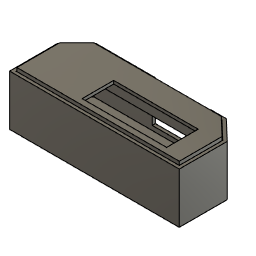
humid_atmega328p v1 (Autodesk Fusion 360 design; units mm, degrees)
Autodesk Fusion 360 part; units mm, degrees
sketch "base" plane through (0, 0, 0) normal (0, 1, 0) x (1, 0, 0)
  line L0 (-25.5013, -7.5251) -> (-25.5013, -7.5251)
  line L1 (26.2751, 6.2603) -> (26.2751, -7.5251)
  line L2 (26.2751, -7.5251) -> (-25.5249, -7.5251)
  line L3 (-25.5249, -7.5251) -> (-25.5249, 6.2605)
  line L4 (-25.5249, 6.2605) -> (-20.01, 11.7751)
  line L5 (-20.01, 11.7751) -> (20.5096, 11.7751)
  line L6 (20.5096, 11.7751) -> (20.5136, 11.771)
  line L7 (20.5136, 11.771) -> (20.5142, 11.771)
  line L8 (20.5142, 11.771) -> (26.2751, 6.2603)
  line L9 (27.2751, 6.6876) -> (27.2751, -8.5251)
  line L10 (27.2751, -8.5251) -> (-26.5249, -8.5251)
  line L11 (-26.5249, -8.5251) -> (-26.5249, 6.6747)
  line L12 (-26.5249, 6.6747) -> (-20.4242, 12.7751)
  line L13 (-20.4242, 12.7751) -> (20.9238, 12.7751)
  line L14 (20.9238, 12.7751) -> (21.2002, 12.4987)
  line L15 (21.2002, 12.4987) -> (27.2751, 6.6876)
  line L16 (20.454, 11.621) -> (26.1251, 6.1963)
  line L17 (26.1251, 6.1963) -> (26.1251, -7.3751)
  line L18 (26.1251, -7.3751) -> (-25.3749, -7.3751)
  line L19 (-25.3749, -7.3751) -> (-25.3749, 6.1983)
  line L20 (-25.3749, 6.1983) -> (-19.9479, 11.6251)
  line L21 (-19.9479, 11.6251) -> (20.4474, 11.6251)
  line L22 (20.4474, 11.6251) -> (20.4515, 11.621)
  line L23 (20.4515, 11.621) -> (20.454, 11.621)
  line L24 (25.2751, 5.8331) -> (25.2751, -6.5251)
  line L25 (25.2751, -6.5251) -> (-24.5249, -6.5251)
  line L26 (-24.5249, -6.5251) -> (-24.5249, 5.8463)
  line L27 (-24.5249, 5.8463) -> (-19.5958, 10.7751)
  line L28 (-19.5958, 10.7751) -> (20.0954, 10.7751)
  line L29 (20.0954, 10.7751) -> (20.0994, 10.771)
  line L30 (20.0994, 10.771) -> (20.1129, 10.771)
  line L31 (20.1129, 10.771) -> (25.2751, 5.8331)
  dimension "d3" = -1
  dimension "d16" = 0.15
  dimension "d17" = 1
extrude "Extrude1" add sketch "base" along normal blind 2 contours L1 L2 L3 L4 L5 L6 L8 | L9 L10 L11 L12 L13 L14 L15 | L16 L17 L18 L19 L20 L21 L22 L23 | L24 L25 L26 L27 L28 L29 L30 L31 makes body 1
extrude "Extrude2" add sketch "base" along normal blind 16 contours L9 L10 L11 L12 L13 L14 L15 bodies 1
extrude "Extrude4" add sketch "base" along normal blind 16 separate body contours L16 L17 L18 L19 L20 L21 L22 L23 makes body 2
extrude "Extrude5" add sketch "base" against normal blind 3 from surface at 16 contours L24 L25 L26 L27 L28 L29 L30 L31 bodies 2
move_body "Move1" bodies 2 to x (1, 0, 0) y (0, 1, 0) z (0, 0, 1) at (0, 1, 0)
extrude "Extrude6" cut 1 faces at (8.6751, 1, 7.0918) along direction (0, 1, 0) blind 7 on bodies 2 bodies 1 2
delete_face "DeleteFace1" 1 faces at (21.108, 10.6667, -12.5908) on bodies 1
sketch "i/o" plane through (0, 0, -12.7751) normal (0, 0, -1) x (-1, 0, 0)
  line L0 (-20.9112, 16) -> (-20.9112, 0)
  line L1 (-20.9112, 0) -> (20.4242, 0)
  line L2 (20.4242, 0) -> (20.4242, 16)
  line L3 (20.4242, 16) -> (-20.9112, 16)
  line L4 (-20.9112, 0) -> (-20.9112, 2) construction
  line L5 (-20.9112, 2) -> (-18.9112, 2) construction
  line L6 (-18.9112, 2) -> (-14.9112, 2) construction
  line L7 (-14.9112, 2) -> (-14.9112, 3.4) construction
  line L8 (-14.9112, 3.4) -> (0.5888, 3.4)
  line L9 (0.5888, 3.4) -> (0.5888, 8.2)
  line L10 (0.5888, 8.2) -> (-14.9112, 8.2)
  line L11 (-14.9112, 8.2) -> (-14.9112, 3.4)
  dimension "d25" = 2
  dimension "d26" = 4
  dimension "d27" = 1.4
  dimension "d28" = 15.5
  dimension "d29" = 4.8
  constraint coincident L0.end L1.start
  constraint coincident L0 L4.end
  constraint perpendicular L1 L4
  constraint perpendicular L4 L5
  constraint parallel L5 L6
  constraint perpendicular L6 L7
  constraint horizontal L8
  constraint vertical L9
  constraint horizontal L10
  constraint vertical L11
  measures "d25" distance of L4.end L5.end
  measures "d26" distance of L5.end L6.end
  measures "d27" distance of L6.end L7.end
  measures "d28" distance of L7.end L8.end
  measures "d29" distance of L7.end L10.end
extrude "Extrude7" cut sketch "i/o" against normal blind 2 contours L8 L9 L10 L11 bodies 1
extrude "Extrude8" add 1 faces at (8.6751, 1, 7.0918) along direction (0, 1, 0) blind 1 on bodies 1 bodies 1
sketch "screen" plane through (0, 17, 0) normal (0, 1, 0) x (-1, 0, 0)
  line L0 (-20.4515, -11.621) -> (-20.4474, -11.6251)
  line L1 (-20.4474, -11.6251) -> (19.9479, -11.6251)
  line L2 (19.9479, -11.6251) -> (25.3749, -6.1983)
  line L3 (25.3749, -6.1983) -> (25.3749, 7.3751)
  line L4 (25.3749, 7.3751) -> (-26.1251, 7.3751)
  line L5 (-26.1251, 7.3751) -> (-26.1251, -6.1963)
  line L6 (-26.1251, -6.1963) -> (-20.454, -11.621)
  line L7 (-20.454, -11.621) -> (-20.4515, -11.621)
  line L8 (-26.1251, 7.3751) -> (-26.1251, 5.5751) construction
  line L9 (-26.1251, 5.5751) -> (-21.5251, 5.5751) construction
  line L10 (-21.5251, 5.5751) -> (4.4749, 5.5751)
  line L11 (4.4749, 5.5751) -> (4.4749, -4.4249)
  line L12 (4.4749, -4.4249) -> (-21.5251, -4.4249)
  line L13 (-21.5251, -4.4249) -> (-21.5251, 5.5751)
  dimension "d34" = 1.8
  dimension "d35" = 4.6
  dimension "d36" = 26
  dimension "d37" = 10
  constraint coincident L4.end L5.start
  constraint perpendicular L4 L8
  constraint perpendicular L5 L9
  constraint horizontal L10
  constraint vertical L11
  constraint horizontal L12
  constraint vertical L13
  measures "d34" distance of L4.end L8.end
  measures "d35" distance of L8.end L9.end
  measures "d36" distance of L9.end L10.end
  measures "d37" distance of L9.end L12.end
extrude "Extrude9" cut sketch "screen" against normal blind 3 contours L10 L11 L12 L13 bodies 2
extrude "Extrude10" cut 1 faces at (4.5779, 8.2, -12.4417) along direction (0, 1, 0) blind 0.5 on bodies 1 bodies 1
extrude "Extrude11" cut 1 faces at (8.6751, 8, 7.0918) along direction (0, 1, 0) blind 1 on bodies 2 bodies 2
extrude "Extrude12" cut 1 faces at (-17.8415, 14, -1.2487) along direction (0, 1, 0) blind 2 on bodies 2 bodies 2
extrude "Extrude13" add 1 faces at (21.5251, 16.6667, -1.0916) along direction (-1, 0, 0) blind 1.2 on bodies 2 bodies 2
extrude "Extrude14" cut 1 faces at (-4.4749, 16.6667, 2.2418) along direction (-1, 0, 0) blind 2 on bodies 2 bodies 2
extrude "Extrude15" cut 1 faces at (14.9112, 6.9333, -12.4417) along direction (1, 0, 0) blind 1 on bodies 1 bodies 1
extrude "Extrude16" cut 1 faces at (-0.5888, 5.1667, -12.4417) along direction (-1, 0, 0) blind 1 on bodies 1 bodies 1
extrude "Extrude17" cut 1 faces at (10.0779, 8.7, -12.4417) along direction (0, 1, 0) blind 8 on bodies 1 bodies 1
extrude "Extrude18" add 1 faces at (8.6751, 9, 7.0918) along direction (0, -1, 0) blind 2 on bodies 2 bodies 2
named bodies: "bottom", "lid"
